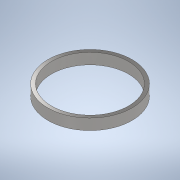
# Autodesk Inventor part: Винт 5x8 2
Saved by Autodesk Inventor 2020 (Build 240168000, 168)
## iProperties
Created: 2021-04-26
Part Number: Винт 5x8 2
Material: Сталь, мягкая
Document SubType Name: Modeling
Designer: lbfas
Density: 7.85 g/cm^3
Appearance: С умеренной полировкой
Author: lbfas
Autodesk Inventor part; units mm, degrees
ref_plane "YZ Plane" through (0, 0, 0) normal (1, 0, 0) x (0, 1, 0)
ref_plane "XZ Plane" through (0, 0, 0) normal (0, 1, 0) x (-1, 0, 0)
ref_plane "XY Plane" through (0, 0, 0) normal (0, 0, 1) x (1, 0, 0)
sketch "Эскиз1" plane through (0, 0, 0) normal (0, 1, 0) x (-1, 0, 0)
  circle A0 centre (0, 0) radius 6
  circle A1 centre (0, 0) radius 5.5
  dimension "d0" = 12
  dimension "d1" = 11
  constraints: 2 centre point, 2 coincident
  measures "d0" diameter of A0
  measures "d1" diameter of A1
extrude "Выдавливание1" add sketch "Эскиз1" along normal blind 1.55
